Autodesk Fusion 360 part; units mm, degrees
(part 9 of 12)
sketch "草图30" plane through (71.5001, 0.0001, 0) normal (1, 0.000001, 0) x (-0.000001, 1, 0)
  line L0 (-74.9988, 0) -> (161.4999, 0)
  line L1 (161.4999, 0) -> (161.4999, 250)
  line L2 (161.4999, 250) -> (-74.9988, 250)
  line L3 (-74.9988, 250) -> (-74.9988, 0)
  line L4 (-64.9988, 15) -> (-69.3289, 12.5)
  line L5 (-69.3289, 12.5) -> (-69.3289, 7.5)
  line L6 (-69.3289, 7.5) -> (-64.9988, 5)
  line L7 (-64.9988, 5) -> (-60.6687, 7.5)
  line L8 (-60.6687, 7.5) -> (-60.6687, 12.5)
  line L9 (-60.6687, 12.5) -> (-64.9988, 15)
  line L10 (-54.3385, 15) -> (-58.6687, 12.5)
  line L11 (-58.6687, 12.5) -> (-58.6687, 7.5)
  line L12 (-58.6687, 7.5) -> (-54.3385, 5)
  line L13 (-54.3385, 5) -> (-50.0084, 7.5)
  line L14 (-50.0084, 7.5) -> (-50.0084, 12.5)
  line L15 (-50.0084, 12.5) -> (-54.3385, 15)
  line L16 (-43.6783, 15) -> (-48.0084, 12.5)
  line L17 (-48.0084, 12.5) -> (-48.0084, 7.5)
  line L18 (-48.0084, 7.5) -> (-43.6783, 5)
  line L19 (-43.6783, 5) -> (-39.3482, 7.5)
  line L20 (-39.3482, 7.5) -> (-39.3482, 12.5)
  line L21 (-39.3482, 12.5) -> (-43.6783, 15)
  line L22 (-33.018, 15) -> (-37.3482, 12.5)
  line L23 (-37.3482, 12.5) -> (-37.3482, 7.5)
  line L24 (-37.3482, 7.5) -> (-33.018, 5)
  line L25 (-33.018, 5) -> (-28.6879, 7.5)
  line L26 (-28.6879, 7.5) -> (-28.6879, 12.5)
  line L27 (-28.6879, 12.5) -> (-33.018, 15)
  line L28 (-22.3578, 15) -> (-26.6879, 12.5)
  line L29 (-26.6879, 12.5) -> (-26.6879, 7.5)
  line L30 (-26.6879, 7.5) -> (-22.3578, 5)
  line L31 (-22.3578, 5) -> (-18.0277, 7.5)
  line L32 (-18.0277, 7.5) -> (-18.0277, 12.5)
  line L33 (-18.0277, 12.5) -> (-22.3578, 15)
  line L34 (-11.6975, 15) -> (-16.0277, 12.5)
  line L35 (-16.0277, 12.5) -> (-16.0277, 7.5)
  line L36 (-16.0277, 7.5) -> (-11.6975, 5)
  line L37 (-11.6975, 5) -> (-7.3674, 7.5)
  line L38 (-7.3674, 7.5) -> (-7.3674, 12.5)
  line L39 (-7.3674, 12.5) -> (-11.6975, 15)
  line L40 (-1.0373, 15) -> (-5.3674, 12.5)
  line L41 (-5.3674, 12.5) -> (-5.3674, 7.5)
  line L42 (-5.3674, 7.5) -> (-1.0373, 5)
  line L43 (-1.0373, 5) -> (3.2929, 7.5)
  line L44 (3.2929, 7.5) -> (3.2929, 12.5)
  line L45 (3.2929, 12.5) -> (-1.0373, 15)
  line L46 (9.623, 15) -> (5.2929, 12.5)
  line L47 (5.2929, 12.5) -> (5.2929, 7.5)
  line L48 (5.2929, 7.5) -> (9.623, 5)
  line L49 (9.623, 5) -> (13.9531, 7.5)
  line L50 (13.9531, 7.5) -> (13.9531, 12.5)
  line L51 (13.9531, 12.5) -> (9.623, 15)
  line L52 (20.2832, 15) -> (15.9531, 12.5)
  line L53 (15.9531, 12.5) -> (15.9531, 7.5)
  line L54 (15.9531, 7.5) -> (20.2832, 5)
  line L55 (20.2832, 5) -> (24.6134, 7.5)
  line L56 (24.6134, 7.5) -> (24.6134, 12.5)
  line L57 (24.6134, 12.5) -> (20.2832, 15)
  line L58 (30.9435, 15) -> (26.6134, 12.5)
  line L59 (26.6134, 12.5) -> (26.6134, 7.5)
  line L60 (26.6134, 7.5) -> (30.9435, 5)
  line L61 (30.9435, 5) -> (35.2736, 7.5)
  line L62 (35.2736, 7.5) -> (35.2736, 12.5)
  line L63 (35.2736, 12.5) -> (30.9435, 15)
  line L64 (41.6037, 15) -> (37.2736, 12.5)
  line L65 (37.2736, 12.5) -> (37.2736, 7.5)
  line L66 (37.2736, 7.5) -> (41.6037, 5)
  line L67 (41.6037, 5) -> (45.9339, 7.5)
  line L68 (45.9339, 7.5) -> (45.9339, 12.5)
  line L69 (45.9339, 12.5) -> (41.6037, 15)
  line L70 (52.264, 15) -> (47.9339, 12.5)
  line L71 (47.9339, 12.5) -> (47.9339, 7.5)
  line L72 (47.9339, 7.5) -> (52.264, 5)
  line L73 (52.264, 5) -> (56.5941, 7.5)
  line L74 (56.5941, 7.5) -> (56.5941, 12.5)
  line L75 (56.5941, 12.5) -> (52.264, 15)
  line L76 (62.9242, 15) -> (58.5941, 12.5)
  line L77 (58.5941, 12.5) -> (58.5941, 7.5)
  line L78 (58.5941, 7.5) -> (62.9242, 5)
  line L79 (62.9242, 5) -> (67.2544, 7.5)
  line L80 (67.2544, 7.5) -> (67.2544, 12.5)
  line L81 (67.2544, 12.5) -> (62.9242, 15)
  line L82 (73.5845, 15) -> (69.2544, 12.5)
  line L83 (69.2544, 12.5) -> (69.2544, 7.5)
  line L84 (69.2544, 7.5) -> (73.5845, 5)
  line L85 (73.5845, 5) -> (77.9146, 7.5)
  line L86 (77.9146, 7.5) -> (77.9146, 12.5)
  line L87 (77.9146, 12.5) -> (73.5845, 15)
  line L88 (84.2448, 15) -> (79.9146, 12.5)
  line L89 (79.9146, 12.5) -> (79.9146, 7.5)
  line L90 (79.9146, 7.5) -> (84.2448, 5)
  line L91 (84.2448, 5) -> (88.5749, 7.5)
  line L92 (88.5749, 7.5) -> (88.5749, 12.5)
  line L93 (88.5749, 12.5) -> (84.2448, 15)
  line L94 (94.905, 15) -> (90.5749, 12.5)
  line L95 (90.5749, 12.5) -> (90.5749, 7.5)
  line L96 (90.5749, 7.5) -> (94.905, 5)
  line L97 (94.905, 5) -> (99.2351, 7.5)
  line L98 (99.2351, 7.5) -> (99.2351, 12.5)
  line L99 (99.2351, 12.5) -> (94.905, 15)
  line L100 (105.5653, 15) -> (101.2351, 12.5)
  line L101 (101.2351, 12.5) -> (101.2351, 7.5)
  line L102 (101.2351, 7.5) -> (105.5653, 5)
  line L103 (105.5653, 5) -> (109.8954, 7.5)
  line L104 (109.8954, 7.5) -> (109.8954, 12.5)
  line L105 (109.8954, 12.5) -> (105.5653, 15)
  line L106 (116.2255, 15) -> (111.8954, 12.5)
  line L107 (111.8954, 12.5) -> (111.8954, 7.5)
  line L108 (111.8954, 7.5) -> (116.2255, 5)
  line L109 (116.2255, 5) -> (120.5556, 7.5)
  line L110 (120.5556, 7.5) -> (120.5556, 12.5)
  line L111 (120.5556, 12.5) -> (116.2255, 15)
  line L112 (126.8858, 15) -> (122.5556, 12.5)
  line L113 (122.5556, 12.5) -> (122.5556, 7.5)
  line L114 (122.5556, 7.5) -> (126.8858, 5)
  line L115 (126.8858, 5) -> (131.2159, 7.5)
  line L116 (131.2159, 7.5) -> (131.2159, 12.5)
  line L117 (131.2159, 12.5) -> (126.8858, 15)
  line L118 (137.546, 15) -> (133.2159, 12.5)
  line L119 (133.2159, 12.5) -> (133.2159, 7.5)
  line L120 (133.2159, 7.5) -> (137.546, 5)
  line L121 (137.546, 5) -> (141.8762, 7.5)
  line L122 (141.8762, 7.5) -> (141.8762, 12.5)
  line L123 (141.8762, 12.5) -> (137.546, 15)
  line L124 (148.2063, 15) -> (143.8762, 12.5)
  line L125 (143.8762, 12.5) -> (143.8762, 7.5)
  line L126 (143.8762, 7.5) -> (148.2063, 5)
  line L127 (148.2063, 5) -> (152.5364, 7.5)
  line L128 (152.5364, 7.5) -> (152.5364, 12.5)
  line L129 (152.5364, 12.5) -> (148.2063, 15)
  line L130 (-59.6687, 24.2321) -> (-63.9988, 21.7321)
  line L131 (-63.9988, 21.7321) -> (-63.9988, 16.7321)
  line L132 (-63.9988, 16.7321) -> (-59.6687, 14.2321)
  line L133 (-59.6687, 14.2321) -> (-55.3385, 16.7321)
  line L134 (-55.3385, 16.7321) -> (-55.3385, 21.7321)
  line L135 (-55.3385, 21.7321) -> (-59.6687, 24.2321)
  line L136 (-49.0084, 24.2321) -> (-53.3385, 21.7321)
  line L137 (-53.3385, 21.7321) -> (-53.3385, 16.7321)
  line L138 (-53.3385, 16.7321) -> (-49.0084, 14.2321)
  line L139 (-49.0084, 14.2321) -> (-44.6783, 16.7321)
  line L140 (-44.6783, 16.7321) -> (-44.6783, 21.7321)
  line L141 (-44.6783, 21.7321) -> (-49.0084, 24.2321)
  line L142 (-38.3482, 24.2321) -> (-42.6783, 21.7321)
  line L143 (-42.6783, 21.7321) -> (-42.6783, 16.7321)
  line L144 (-42.6783, 16.7321) -> (-38.3482, 14.2321)
  line L145 (-38.3482, 14.2321) -> (-34.018, 16.7321)
  line L146 (-34.018, 16.7321) -> (-34.018, 21.7321)
  line L147 (-34.018, 21.7321) -> (-38.3482, 24.2321)
  line L148 (-27.6879, 24.2321) -> (-32.018, 21.7321)
  line L149 (-32.018, 21.7321) -> (-32.018, 16.7321)
  line L150 (-32.018, 16.7321) -> (-27.6879, 14.2321)
  line L151 (-27.6879, 14.2321) -> (-23.3578, 16.7321)
  line L152 (-23.3578, 16.7321) -> (-23.3578, 21.7321)
  line L153 (-23.3578, 21.7321) -> (-27.6879, 24.2321)
  line L154 (-17.0277, 24.2321) -> (-21.3578, 21.7321)
  line L155 (-21.3578, 21.7321) -> (-21.3578, 16.7321)
  line L156 (-21.3578, 16.7321) -> (-17.0277, 14.2321)
  line L157 (-17.0277, 14.2321) -> (-12.6975, 16.7321)
  line L158 (-12.6975, 16.7321) -> (-12.6975, 21.7321)
  line L159 (-12.6975, 21.7321) -> (-17.0277, 24.2321)
  line L160 (-6.3674, 24.2321) -> (-10.6975, 21.7321)
  line L161 (-10.6975, 21.7321) -> (-10.6975, 16.7321)
  line L162 (-10.6975, 16.7321) -> (-6.3674, 14.2321)
  line L163 (-6.3674, 14.2321) -> (-2.0373, 16.7321)
  line L164 (-2.0373, 16.7321) -> (-2.0373, 21.7321)
  line L165 (-2.0373, 21.7321) -> (-6.3674, 24.2321)
  line L166 (4.2929, 24.2321) -> (-0.0373, 21.7321)
  line L167 (-0.0373, 21.7321) -> (-0.0373, 16.7321)
  line L168 (-0.0373, 16.7321) -> (4.2929, 14.2321)
  line L169 (4.2929, 14.2321) -> (8.623, 16.7321)
  line L170 (8.623, 16.7321) -> (8.623, 21.7321)
  line L171 (8.623, 21.7321) -> (4.2929, 24.2321)
  line L172 (14.9531, 24.2321) -> (10.623, 21.7321)
  line L173 (10.623, 21.7321) -> (10.623, 16.7321)
  line L174 (10.623, 16.7321) -> (14.9531, 14.2321)
  line L175 (14.9531, 14.2321) -> (19.2832, 16.7321)
  line L176 (19.2832, 16.7321) -> (19.2832, 21.7321)
  line L177 (19.2832, 21.7321) -> (14.9531, 24.2321)
  line L178 (25.6134, 24.2321) -> (21.2832, 21.7321)
  line L179 (21.2832, 21.7321) -> (21.2832, 16.7321)
  line L180 (21.2832, 16.7321) -> (25.6134, 14.2321)
  line L181 (25.6134, 14.2321) -> (29.9435, 16.7321)
  line L182 (29.9435, 16.7321) -> (29.9435, 21.7321)
  line L183 (29.9435, 21.7321) -> (25.6134, 24.2321)
  line L184 (36.2736, 24.2321) -> (31.9435, 21.7321)
  line L185 (31.9435, 21.7321) -> (31.9435, 16.7321)
  line L186 (31.9435, 16.7321) -> (36.2736, 14.2321)
  line L187 (36.2736, 14.2321) -> (40.6037, 16.7321)
  line L188 (40.6037, 16.7321) -> (40.6037, 21.7321)
  line L189 (40.6037, 21.7321) -> (36.2736, 24.2321)
  line L190 (46.9339, 24.2321) -> (42.6037, 21.7321)
  line L191 (42.6037, 21.7321) -> (42.6037, 16.7321)
  line L192 (42.6037, 16.7321) -> (46.9339, 14.2321)
  line L193 (46.9339, 14.2321) -> (51.264, 16.7321)
  line L194 (51.264, 16.7321) -> (51.264, 21.7321)
  line L195 (51.264, 21.7321) -> (46.9339, 24.2321)
  line L196 (57.5941, 24.2321) -> (53.264, 21.7321)
  line L197 (53.264, 21.7321) -> (53.264, 16.7321)
  line L198 (53.264, 16.7321) -> (57.5941, 14.2321)
  line L199 (57.5941, 14.2321) -> (61.9242, 16.7321)
  line L200 (61.9242, 16.7321) -> (61.9242, 21.7321)
  line L201 (61.9242, 21.7321) -> (57.5941, 24.2321)
  line L202 (68.2544, 24.2321) -> (63.9242, 21.7321)
  line L203 (63.9242, 21.7321) -> (63.9242, 16.7321)
  line L204 (63.9242, 16.7321) -> (68.2544, 14.2321)
  line L205 (68.2544, 14.2321) -> (72.5845, 16.7321)
  line L206 (72.5845, 16.7321) -> (72.5845, 21.7321)
  line L207 (72.5845, 21.7321) -> (68.2544, 24.2321)
  line L208 (78.9146, 24.2321) -> (74.5845, 21.7321)
  line L209 (74.5845, 21.7321) -> (74.5845, 16.7321)
  line L210 (74.5845, 16.7321) -> (78.9146, 14.2321)
  line L211 (78.9146, 14.2321) -> (83.2448, 16.7321)
  line L212 (83.2448, 16.7321) -> (83.2448, 21.7321)
  line L213 (83.2448, 21.7321) -> (78.9146, 24.2321)
  line L214 (89.5749, 24.2321) -> (85.2448, 21.7321)
  line L215 (85.2448, 21.7321) -> (85.2448, 16.7321)
  line L216 (85.2448, 16.7321) -> (89.5749, 14.2321)
  line L217 (89.5749, 14.2321) -> (93.905, 16.7321)
  line L218 (93.905, 16.7321) -> (93.905, 21.7321)
  line L219 (93.905, 21.7321) -> (89.5749, 24.2321)
  line L220 (100.2351, 24.2321) -> (95.905, 21.7321)
  line L221 (95.905, 21.7321) -> (95.905, 16.7321)
  line L222 (95.905, 16.7321) -> (100.2351, 14.2321)
  line L223 (100.2351, 14.2321) -> (104.5653, 16.7321)
  line L224 (104.5653, 16.7321) -> (104.5653, 21.7321)
  line L225 (104.5653, 21.7321) -> (100.2351, 24.2321)
  line L226 (110.8954, 24.2321) -> (106.5653, 21.7321)
  line L227 (106.5653, 21.7321) -> (106.5653, 16.7321)
  line L228 (106.5653, 16.7321) -> (110.8954, 14.2321)
  line L229 (110.8954, 14.2321) -> (115.2255, 16.7321)
  line L230 (115.2255, 16.7321) -> (115.2255, 21.7321)
  line L231 (115.2255, 21.7321) -> (110.8954, 24.2321)
  line L232 (121.5556, 24.2321) -> (117.2255, 21.7321)
  line L233 (117.2255, 21.7321) -> (117.2255, 16.7321)
  line L234 (117.2255, 16.7321) -> (121.5556, 14.2321)
  line L235 (121.5556, 14.2321) -> (125.8858, 16.7321)
  line L236 (125.8858, 16.7321) -> (125.8858, 21.7321)
  line L237 (125.8858, 21.7321) -> (121.5556, 24.2321)
  line L238 (132.2159, 24.2321) -> (127.8858, 21.7321)
  line L239 (127.8858, 21.7321) -> (127.8858, 16.7321)
  line L240 (127.8858, 16.7321) -> (132.2159, 14.2321)
  line L241 (132.2159, 14.2321) -> (136.546, 16.7321)
  line L242 (136.546, 16.7321) -> (136.546, 21.7321)
  line L243 (136.546, 21.7321) -> (132.2159, 24.2321)
  line L244 (142.8762, 24.2321) -> (138.546, 21.7321)
  line L245 (138.546, 21.7321) -> (138.546, 16.7321)
  line L246 (138.546, 16.7321) -> (142.8762, 14.2321)
  line L247 (142.8762, 14.2321) -> (147.2063, 16.7321)
  line L248 (147.2063, 16.7321) -> (147.2063, 21.7321)
  line L249 (147.2063, 21.7321) -> (142.8762, 24.2321)
  line L250 (-64.9988, 33.4641) -> (-69.3289, 30.9641)
  line L251 (-69.3289, 30.9641) -> (-69.3289, 25.9641)
  line L252 (-69.3289, 25.9641) -> (-64.9988, 23.4641)
  line L253 (-64.9988, 23.4641) -> (-60.6687, 25.9641)
  line L254 (-60.6687, 25.9641) -> (-60.6687, 30.9641)
  line L255 (-60.6687, 30.9641) -> (-64.9988, 33.4641)
  line L256 (-54.3385, 33.4641) -> (-58.6687, 30.9641)
  line L257 (-58.6687, 30.9641) -> (-58.6687, 25.9641)
  line L258 (-58.6687, 25.9641) -> (-54.3385, 23.4641)
  line L259 (-54.3385, 23.4641) -> (-50.0084, 25.9641)
  line L260 (-50.0084, 25.9641) -> (-50.0084, 30.9641)
  line L261 (-50.0084, 30.9641) -> (-54.3385, 33.4641)
  line L262 (-43.6783, 33.4641) -> (-48.0084, 30.9641)
  line L263 (-48.0084, 30.9641) -> (-48.0084, 25.9641)
  line L264 (-48.0084, 25.9641) -> (-43.6783, 23.4641)
  line L265 (-43.6783, 23.4641) -> (-39.3482, 25.9641)
  line L266 (-39.3482, 25.9641) -> (-39.3482, 30.9641)
  line L267 (-39.3482, 30.9641) -> (-43.6783, 33.4641)
  line L268 (-33.018, 33.4641) -> (-37.3482, 30.9641)
  line L269 (-37.3482, 30.9641) -> (-37.3482, 25.9641)
  line L270 (-37.3482, 25.9641) -> (-33.018, 23.4641)
  line L271 (-33.018, 23.4641) -> (-28.6879, 25.9641)
  line L272 (-28.6879, 25.9641) -> (-28.6879, 30.9641)
  line L273 (-28.6879, 30.9641) -> (-33.018, 33.4641)
  line L274 (-22.3578, 33.4641) -> (-26.6879, 30.9641)
  line L275 (-26.6879, 30.9641) -> (-26.6879, 25.9641)
  line L276 (-26.6879, 25.9641) -> (-22.3578, 23.4641)
  line L277 (-22.3578, 23.4641) -> (-18.0277, 25.9641)
  line L278 (-18.0277, 25.9641) -> (-18.0277, 30.9641)
  line L279 (-18.0277, 30.9641) -> (-22.3578, 33.4641)
  line L280 (-11.6975, 33.4641) -> (-16.0277, 30.9641)
  line L281 (-16.0277, 30.9641) -> (-16.0277, 25.9641)
  line L282 (-16.0277, 25.9641) -> (-11.6975, 23.4641)
  line L283 (-11.6975, 23.4641) -> (-7.3674, 25.9641)
  line L284 (-7.3674, 25.9641) -> (-7.3674, 30.9641)
  line L285 (-7.3674, 30.9641) -> (-11.6975, 33.4641)
  line L286 (-1.0373, 33.4641) -> (-5.3674, 30.9641)
  line L287 (-5.3674, 30.9641) -> (-5.3674, 25.9641)
  line L288 (-5.3674, 25.9641) -> (-1.0373, 23.4641)
  line L289 (-1.0373, 23.4641) -> (3.2929, 25.9641)
  line L290 (3.2929, 25.9641) -> (3.2929, 30.9641)
  line L291 (3.2929, 30.9641) -> (-1.0373, 33.4641)
  line L292 (9.623, 33.4641) -> (5.2929, 30.9641)
  line L293 (5.2929, 30.9641) -> (5.2929, 25.9641)
  line L294 (5.2929, 25.9641) -> (9.623, 23.4641)
  line L295 (9.623, 23.4641) -> (13.9531, 25.9641)
  line L296 (13.9531, 25.9641) -> (13.9531, 30.9641)
  line L297 (13.9531, 30.9641) -> (9.623, 33.4641)
  line L298 (20.2832, 33.4641) -> (15.9531, 30.9641)
  line L299 (15.9531, 30.9641) -> (15.9531, 25.9641)
  line L300 (15.9531, 25.9641) -> (20.2832, 23.4641)
  line L301 (20.2832, 23.4641) -> (24.6134, 25.9641)
  line L302 (24.6134, 25.9641) -> (24.6134, 30.9641)
  line L303 (24.6134, 30.9641) -> (20.2832, 33.4641)
  line L304 (30.9435, 33.4641) -> (26.6134, 30.9641)
  line L305 (26.6134, 30.9641) -> (26.6134, 25.9641)
  line L306 (26.6134, 25.9641) -> (30.9435, 23.4641)
  line L307 (30.9435, 23.4641) -> (35.2736, 25.9641)
  line L308 (35.2736, 25.9641) -> (35.2736, 30.9641)
  line L309 (35.2736, 30.9641) -> (30.9435, 33.4641)
  line L310 (41.6037, 33.4641) -> (37.2736, 30.9641)
  line L311 (37.2736, 30.9641) -> (37.2736, 25.9641)
  line L312 (37.2736, 25.9641) -> (41.6037, 23.4641)
  line L313 (41.6037, 23.4641) -> (45.9339, 25.9641)
  line L314 (45.9339, 25.9641) -> (45.9339, 30.9641)
  line L315 (45.9339, 30.9641) -> (41.6037, 33.4641)
  line L316 (52.264, 33.4641) -> (47.9339, 30.9641)
  line L317 (47.9339, 30.9641) -> (47.9339, 25.9641)
  line L318 (47.9339, 25.9641) -> (52.264, 23.4641)
  line L319 (52.264, 23.4641) -> (56.5941, 25.9641)
  line L320 (56.5941, 25.9641) -> (56.5941, 30.9641)
  line L321 (56.5941, 30.9641) -> (52.264, 33.4641)
  line L322 (62.9242, 33.4641) -> (58.5941, 30.9641)
  line L323 (58.5941, 30.9641) -> (58.5941, 25.9641)
  line L324 (58.5941, 25.9641) -> (62.9242, 23.4641)
  line L325 (62.9242, 23.4641) -> (67.2544, 25.9641)
  line L326 (67.2544, 25.9641) -> (67.2544, 30.9641)
  line L327 (67.2544, 30.9641) -> (62.9242, 33.4641)
  line L328 (73.5845, 33.4641) -> (69.2544, 30.9641)
  line L329 (69.2544, 30.9641) -> (69.2544, 25.9641)
  line L330 (69.2544, 25.9641) -> (73.5845, 23.4641)
  line L331 (73.5845, 23.4641) -> (77.9146, 25.9641)
  line L332 (77.9146, 25.9641) -> (77.9146, 30.9641)
  line L333 (77.9146, 30.9641) -> (73.5845, 33.4641)
  line L334 (84.2448, 33.4641) -> (79.9146, 30.9641)
  line L335 (79.9146, 30.9641) -> (79.9146, 25.9641)
  line L336 (79.9146, 25.9641) -> (84.2448, 23.4641)
  line L337 (84.2448, 23.4641) -> (88.5749, 25.9641)
  line L338 (88.5749, 25.9641) -> (88.5749, 30.9641)
  line L339 (88.5749, 30.9641) -> (84.2448, 33.4641)
  line L340 (94.905, 33.4641) -> (90.5749, 30.9641)
  line L341 (90.5749, 30.9641) -> (90.5749, 25.9641)
  line L342 (90.5749, 25.9641) -> (94.905, 23.4641)
  line L343 (94.905, 23.4641) -> (99.2351, 25.9641)
  line L344 (99.2351, 25.9641) -> (99.2351, 30.9641)
  line L345 (99.2351, 30.9641) -> (94.905, 33.4641)
  line L346 (105.5653, 33.4641) -> (101.2351, 30.9641)
  line L347 (101.2351, 30.9641) -> (101.2351, 25.9641)
  line L348 (101.2351, 25.9641) -> (105.5653, 23.4641)
  line L349 (105.5653, 23.4641) -> (109.8954, 25.9641)
  line L350 (109.8954, 25.9641) -> (109.8954, 30.9641)
  line L351 (109.8954, 30.9641) -> (105.5653, 33.4641)
  line L352 (116.2255, 33.4641) -> (111.8954, 30.9641)
  line L353 (111.8954, 30.9641) -> (111.8954, 25.9641)
  line L354 (111.8954, 25.9641) -> (116.2255, 23.4641)
  line L355 (116.2255, 23.4641) -> (120.5556, 25.9641)
  line L356 (120.5556, 25.9641) -> (120.5556, 30.9641)
  line L357 (120.5556, 30.9641) -> (116.2255, 33.4641)
  line L358 (126.8858, 33.4641) -> (122.5556, 30.9641)
  line L359 (122.5556, 30.9641) -> (122.5556, 25.9641)
  line L360 (122.5556, 25.9641) -> (126.8858, 23.4641)
  line L361 (126.8858, 23.4641) -> (131.2159, 25.9641)
  line L362 (131.2159, 25.9641) -> (131.2159, 30.9641)
  line L363 (131.2159, 30.9641) -> (126.8858, 33.4641)
  line L364 (137.546, 33.4641) -> (133.2159, 30.9641)
  line L365 (133.2159, 30.9641) -> (133.2159, 25.9641)
  line L366 (133.2159, 25.9641) -> (137.546, 23.4641)
  line L367 (137.546, 23.4641) -> (141.8762, 25.9641)
  line L368 (141.8762, 25.9641) -> (141.8762, 30.9641)
  line L369 (141.8762, 30.9641) -> (137.546, 33.4641)
  line L370 (148.2063, 33.4641) -> (143.8762, 30.9641)
  line L371 (143.8762, 30.9641) -> (143.8762, 25.9641)
  line L372 (143.8762, 25.9641) -> (148.2063, 23.4641)
  line L373 (148.2063, 23.4641) -> (152.5364, 25.9641)
  line L374 (152.5364, 25.9641) -> (152.5364, 30.9641)
  line L375 (152.5364, 30.9641) -> (148.2063, 33.4641)
  line L376 (-59.6687, 42.6962) -> (-63.9988, 40.1962)
  line L377 (-63.9988, 40.1962) -> (-63.9988, 35.1962)
  line L378 (-63.9988, 35.1962) -> (-59.6687, 32.6962)
  line L379 (-59.6687, 32.6962) -> (-55.3385, 35.1962)
  line L380 (-55.3385, 35.1962) -> (-55.3385, 40.1962)
  line L381 (-55.3385, 40.1962) -> (-59.6687, 42.6962)
  line L382 (-49.0084, 42.6962) -> (-53.3385, 40.1962)
  line L383 (-53.3385, 40.1962) -> (-53.3385, 35.1962)
  line L384 (-53.3385, 35.1962) -> (-49.0084, 32.6962)
  line L385 (-49.0084, 32.6962) -> (-44.6783, 35.1962)
  line L386 (-44.6783, 35.1962) -> (-44.6783, 40.1962)
  line L387 (-44.6783, 40.1962) -> (-49.0084, 42.6962)
  line L388 (-38.3482, 42.6962) -> (-42.6783, 40.1962)
  line L389 (-42.6783, 40.1962) -> (-42.6783, 35.1962)
  line L390 (-42.6783, 35.1962) -> (-38.3482, 32.6962)
  line L391 (-38.3482, 32.6962) -> (-34.018, 35.1962)
  line L392 (-34.018, 35.1962) -> (-34.018, 40.1962)
  line L393 (-34.018, 40.1962) -> (-38.3482, 42.6962)
  line L394 (-27.6879, 42.6962) -> (-32.018, 40.1962)
  line L395 (-32.018, 40.1962) -> (-32.018, 35.1962)
  line L396 (-32.018, 35.1962) -> (-27.6879, 32.6962)
  line L397 (-27.6879, 32.6962) -> (-23.3578, 35.1962)
  line L398 (-23.3578, 35.1962) -> (-23.3578, 40.1962)
  line L399 (-23.3578, 40.1962) -> (-27.6879, 42.6962)
  line L400 (-17.0277, 42.6962) -> (-21.3578, 40.1962)
  line L401 (-21.3578, 40.1962) -> (-21.3578, 35.1962)
  line L402 (-21.3578, 35.1962) -> (-17.0277, 32.6962)
  line L403 (-17.0277, 32.6962) -> (-12.6975, 35.1962)
  line L404 (-12.6975, 35.1962) -> (-12.6975, 40.1962)
  line L405 (-12.6975, 40.1962) -> (-17.0277, 42.6962)
  line L406 (-6.3674, 42.6962) -> (-10.6975, 40.1962)
  line L407 (-10.6975, 40.1962) -> (-10.6975, 35.1962)
  line L408 (-10.6975, 35.1962) -> (-6.3674, 32.6962)
  line L409 (-6.3674, 32.6962) -> (-2.0373, 35.1962)
  line L410 (-2.0373, 35.1962) -> (-2.0373, 40.1962)
  line L411 (-2.0373, 40.1962) -> (-6.3674, 42.6962)
  line L412 (4.2929, 42.6962) -> (-0.0373, 40.1962)
  line L413 (-0.0373, 40.1962) -> (-0.0373, 35.1962)
  line L414 (-0.0373, 35.1962) -> (4.2929, 32.6962)
  line L415 (4.2929, 32.6962) -> (8.623, 35.1962)
  line L416 (8.623, 35.1962) -> (8.623, 40.1962)
  line L417 (8.623, 40.1962) -> (4.2929, 42.6962)
  line L418 (14.9531, 42.6962) -> (10.623, 40.1962)
  line L419 (10.623, 40.1962) -> (10.623, 35.1962)
  line L420 (10.623, 35.1962) -> (14.9531, 32.6962)
  line L421 (14.9531, 32.6962) -> (19.2832, 35.1962)
  line L422 (19.2832, 35.1962) -> (19.2832, 40.1962)
  line L423 (19.2832, 40.1962) -> (14.9531, 42.6962)
  line L424 (25.6134, 42.6962) -> (21.2832, 40.1962)
  line L425 (21.2832, 40.1962) -> (21.2832, 35.1962)
  line L426 (21.2832, 35.1962) -> (25.6134, 32.6962)
  line L427 (25.6134, 32.6962) -> (29.9435, 35.1962)
  line L428 (29.9435, 35.1962) -> (29.9435, 40.1962)
  line L429 (29.9435, 40.1962) -> (25.6134, 42.6962)
  line L430 (36.2736, 42.6962) -> (31.9435, 40.1962)
  line L431 (31.9435, 40.1962) -> (31.9435, 35.1962)
  line L432 (31.9435, 35.1962) -> (36.2736, 32.6962)
  line L433 (36.2736, 32.6962) -> (40.6037, 35.1962)
  line L434 (40.6037, 35.1962) -> (40.6037, 40.1962)
  line L435 (40.6037, 40.1962) -> (36.2736, 42.6962)
  line L436 (46.9339, 42.6962) -> (42.6037, 40.1962)
  line L437 (42.6037, 40.1962) -> (42.6037, 35.1962)
  line L438 (42.6037, 35.1962) -> (46.9339, 32.6962)
  line L439 (46.9339, 32.6962) -> (51.264, 35.1962)
  line L440 (51.264, 35.1962) -> (51.264, 40.1962)
  line L441 (51.264, 40.1962) -> (46.9339, 42.6962)
  line L442 (57.5941, 42.6962) -> (53.264, 40.1962)
  line L443 (53.264, 40.1962) -> (53.264, 35.1962)
  line L444 (53.264, 35.1962) -> (57.5941, 32.6962)
  line L445 (57.5941, 32.6962) -> (61.9242, 35.1962)
  line L446 (61.9242, 35.1962) -> (61.9242, 40.1962)
  line L447 (61.9242, 40.1962) -> (57.5941, 42.6962)
  line L448 (68.2544, 42.6962) -> (63.9242, 40.1962)
  line L449 (63.9242, 40.1962) -> (63.9242, 35.1962)
  line L450 (63.9242, 35.1962) -> (68.2544, 32.6962)
  line L451 (68.2544, 32.6962) -> (72.5845, 35.1962)
  line L452 (72.5845, 35.1962) -> (72.5845, 40.1962)
  line L453 (72.5845, 40.1962) -> (68.2544, 42.6962)
  line L454 (78.9146, 42.6962) -> (74.5845, 40.1962)
  line L455 (74.5845, 40.1962) -> (74.5845, 35.1962)
  line L456 (74.5845, 35.1962) -> (78.9146, 32.6962)
  line L457 (78.9146, 32.6962) -> (83.2448, 35.1962)
  line L458 (83.2448, 35.1962) -> (83.2448, 40.1962)
  line L459 (83.2448, 40.1962) -> (78.9146, 42.6962)
  line L460 (89.5749, 42.6962) -> (85.2448, 40.1962)
  line L461 (85.2448, 40.1962) -> (85.2448, 35.1962)
  line L462 (85.2448, 35.1962) -> (89.5749, 32.6962)
  line L463 (89.5749, 32.6962) -> (93.905, 35.1962)
  line L464 (93.905, 35.1962) -> (93.905, 40.1962)
  line L465 (93.905, 40.1962) -> (89.5749, 42.6962)
  line L466 (100.2351, 42.6962) -> (95.905, 40.1962)
  line L467 (95.905, 40.1962) -> (95.905, 35.1962)
  line L468 (95.905, 35.1962) -> (100.2351, 32.6962)
  line L469 (100.2351, 32.6962) -> (104.5653, 35.1962)
  line L470 (104.5653, 35.1962) -> (104.5653, 40.1962)
  line L471 (104.5653, 40.1962) -> (100.2351, 42.6962)
  line L472 (110.8954, 42.6962) -> (106.5653, 40.1962)
  line L473 (106.5653, 40.1962) -> (106.5653, 35.1962)
  line L474 (106.5653, 35.1962) -> (110.8954, 32.6962)
  line L475 (110.8954, 32.6962) -> (115.2255, 35.1962)
  line L476 (115.2255, 35.1962) -> (115.2255, 40.1962)
  line L477 (115.2255, 40.1962) -> (110.8954, 42.6962)
  line L478 (121.5556, 42.6962) -> (117.2255, 40.1962)
  line L479 (117.2255, 40.1962) -> (117.2255, 35.1962)
  line L480 (117.2255, 35.1962) -> (121.5556, 32.6962)
  line L481 (121.5556, 32.6962) -> (125.8858, 35.1962)
  line L482 (125.8858, 35.1962) -> (125.8858, 40.1962)
  line L483 (125.8858, 40.1962) -> (121.5556, 42.6962)
  line L484 (132.2159, 42.6962) -> (127.8858, 40.1962)
  line L485 (127.8858, 40.1962) -> (127.8858, 35.1962)
  line L486 (127.8858, 35.1962) -> (132.2159, 32.6962)
  line L487 (132.2159, 32.6962) -> (136.546, 35.1962)
  line L488 (136.546, 35.1962) -> (136.546, 40.1962)
  line L489 (136.546, 40.1962) -> (132.2159, 42.6962)
  line L490 (142.8762, 42.6962) -> (138.546, 40.1962)
  line L491 (138.546, 40.1962) -> (138.546, 35.1962)
  line L492 (138.546, 35.1962) -> (142.8762, 32.6962)
  line L493 (142.8762, 32.6962) -> (147.2063, 35.1962)
  line L494 (147.2063, 35.1962) -> (147.2063, 40.1962)
  line L495 (147.2063, 40.1962) -> (142.8762, 42.6962)
  line L496 (-64.9988, 51.9282) -> (-69.3289, 49.4282)
  line L497 (-69.3289, 49.4282) -> (-69.3289, 44.4282)
  line L498 (-69.3289, 44.4282) -> (-64.9988, 41.9282)
  line L499 (-64.9988, 41.9282) -> (-60.6687, 44.4282)
  line L500 (-60.6687, 44.4282) -> (-60.6687, 49.4282)
  line L501 (-60.6687, 49.4282) -> (-64.9988, 51.9282)
  line L502 (-54.3385, 51.9282) -> (-58.6687, 49.4282)
  line L503 (-58.6687, 49.4282) -> (-58.6687, 44.4282)
  line L504 (-58.6687, 44.4282) -> (-54.3385, 41.9282)
  line L505 (-54.3385, 41.9282) -> (-50.0084, 44.4282)
  line L506 (-50.0084, 44.4282) -> (-50.0084, 49.4282)
  line L507 (-50.0084, 49.4282) -> (-54.3385, 51.9282)
  line L508 (-43.6783, 51.9282) -> (-48.0084, 49.4282)
  line L509 (-48.0084, 49.4282) -> (-48.0084, 44.4282)
  line L510 (-48.0084, 44.4282) -> (-43.6783, 41.9282)
  line L511 (-43.6783, 41.9282) -> (-39.3482, 44.4282)
  line L512 (-39.3482, 44.4282) -> (-39.3482, 49.4282)
  line L513 (-39.3482, 49.4282) -> (-43.6783, 51.9282)
  line L514 (-33.018, 51.9282) -> (-37.3482, 49.4282)
  line L515 (-37.3482, 49.4282) -> (-37.3482, 44.4282)
  line L516 (-37.3482, 44.4282) -> (-33.018, 41.9282)
  line L517 (-33.018, 41.9282) -> (-28.6879, 44.4282)
  line L518 (-28.6879, 44.4282) -> (-28.6879, 49.4282)
  line L519 (-28.6879, 49.4282) -> (-33.018, 51.9282)
  line L520 (-22.3578, 51.9282) -> (-26.6879, 49.4282)
  line L521 (-26.6879, 49.4282) -> (-26.6879, 44.4282)
  line L522 (-26.6879, 44.4282) -> (-22.3578, 41.9282)
  line L523 (-22.3578, 41.9282) -> (-18.0277, 44.4282)
  line L524 (-18.0277, 44.4282) -> (-18.0277, 49.4282)
  line L525 (-18.0277, 49.4282) -> (-22.3578, 51.9282)
  line L526 (-11.6975, 51.9282) -> (-16.0277, 49.4282)
  line L527 (-16.0277, 49.4282) -> (-16.0277, 44.4282)
  line L528 (-16.0277, 44.4282) -> (-11.6975, 41.9282)
  line L529 (-11.6975, 41.9282) -> (-7.3674, 44.4282)
  line L530 (-7.3674, 44.4282) -> (-7.3674, 49.4282)
  line L531 (-7.3674, 49.4282) -> (-11.6975, 51.9282)
  line L532 (-1.0373, 51.9282) -> (-5.3674, 49.4282)
  line L533 (-5.3674, 49.4282) -> (-5.3674, 44.4282)
  line L534 (-5.3674, 44.4282) -> (-1.0373, 41.9282)
  line L535 (-1.0373, 41.9282) -> (3.2929, 44.4282)
  line L536 (3.2929, 44.4282) -> (3.2929, 49.4282)
  line L537 (3.2929, 49.4282) -> (-1.0373, 51.9282)
  line L538 (9.623, 51.9282) -> (5.2929, 49.4282)
  line L539 (5.2929, 49.4282) -> (5.2929, 44.4282)
  line L540 (5.2929, 44.4282) -> (9.623, 41.9282)
  line L541 (9.623, 41.9282) -> (13.9531, 44.4282)
  line L542 (13.9531, 44.4282) -> (13.9531, 49.4282)
  line L543 (13.9531, 49.4282) -> (9.623, 51.9282)
  line L544 (20.2832, 51.9282) -> (15.9531, 49.4282)
  line L545 (15.9531, 49.4282) -> (15.9531, 44.4282)
  line L546 (15.9531, 44.4282) -> (20.2832, 41.9282)
  line L547 (20.2832, 41.9282) -> (24.6134, 44.4282)
  line L548 (24.6134, 44.4282) -> (24.6134, 49.4282)
  line L549 (24.6134, 49.4282) -> (20.2832, 51.9282)
  line L550 (30.9435, 51.9282) -> (26.6134, 49.4282)
  line L551 (26.6134, 49.4282) -> (26.6134, 44.4282)
  line L552 (26.6134, 44.4282) -> (30.9435, 41.9282)
  line L553 (30.9435, 41.9282) -> (35.2736, 44.4282)
  line L554 (35.2736, 44.4282) -> (35.2736, 49.4282)
  line L555 (35.2736, 49.4282) -> (30.9435, 51.9282)
  line L556 (41.6037, 51.9282) -> (37.2736, 49.4282)
  line L557 (37.2736, 49.4282) -> (37.2736, 44.4282)
  line L558 (37.2736, 44.4282) -> (41.6037, 41.9282)
  line L559 (41.6037, 41.9282) -> (45.9339, 44.4282)
  line L560 (45.9339, 44.4282) -> (45.9339, 49.4282)
  line L561 (45.9339, 49.4282) -> (41.6037, 51.9282)
  line L562 (52.264, 51.9282) -> (47.9339, 49.4282)
  line L563 (47.9339, 49.4282) -> (47.9339, 44.4282)
  line L564 (47.9339, 44.4282) -> (52.264, 41.9282)
  line L565 (52.264, 41.9282) -> (56.5941, 44.4282)
  line L566 (56.5941, 44.4282) -> (56.5941, 49.4282)
  line L567 (56.5941, 49.4282) -> (52.264, 51.9282)
  line L568 (62.9242, 51.9282) -> (58.5941, 49.4282)
  line L569 (58.5941, 49.4282) -> (58.5941, 44.4282)
  line L570 (58.5941, 44.4282) -> (62.9242, 41.9282)
  line L571 (62.9242, 41.9282) -> (67.2544, 44.4282)
  line L572 (67.2544, 44.4282) -> (67.2544, 49.4282)
  line L573 (67.2544, 49.4282) -> (62.9242, 51.9282)
  line L574 (73.5845, 51.9282) -> (69.2544, 49.4282)
  line L575 (69.2544, 49.4282) -> (69.2544, 44.4282)
  line L576 (69.2544, 44.4282) -> (73.5845, 41.9282)
  line L577 (73.5845, 41.9282) -> (77.9146, 44.4282)
  line L578 (77.9146, 44.4282) -> (77.9146, 49.4282)
  line L579 (77.9146, 49.4282) -> (73.5845, 51.9282)
  line L580 (84.2448, 51.9282) -> (79.9146, 49.4282)
  line L581 (79.9146, 49.4282) -> (79.9146, 44.4282)
  line L582 (79.9146, 44.4282) -> (84.2448, 41.9282)
  line L583 (84.2448, 41.9282) -> (88.5749, 44.4282)
  line L584 (88.5749, 44.4282) -> (88.5749, 49.4282)
  line L585 (88.5749, 49.4282) -> (84.2448, 51.9282)
  line L586 (94.905, 51.9282) -> (90.5749, 49.4282)
  line L587 (90.5749, 49.4282) -> (90.5749, 44.4282)
  line L588 (90.5749, 44.4282) -> (94.905, 41.9282)
  line L589 (94.905, 41.9282) -> (99.2351, 44.4282)
  line L590 (99.2351, 44.4282) -> (99.2351, 49.4282)
  line L591 (99.2351, 49.4282) -> (94.905, 51.9282)
  line L592 (105.5653, 51.9282) -> (101.2351, 49.4282)
  line L593 (101.2351, 49.4282) -> (101.2351, 44.4282)
  line L594 (101.2351, 44.4282) -> (105.5653, 41.9282)
  line L595 (105.5653, 41.9282) -> (109.8954, 44.4282)
  line L596 (109.8954, 44.4282) -> (109.8954, 49.4282)
  line L597 (109.8954, 49.4282) -> (105.5653, 51.9282)
  line L598 (116.2255, 51.9282) -> (111.8954, 49.4282)
  line L599 (111.8954, 49.4282) -> (111.8954, 44.4282)
  line L600 (111.8954, 44.4282) -> (116.2255, 41.9282)
  line L601 (116.2255, 41.9282) -> (120.5556, 44.4282)
  line L602 (120.5556, 44.4282) -> (120.5556, 49.4282)
  line L603 (120.5556, 49.4282) -> (116.2255, 51.9282)
  line L604 (126.8858, 51.9282) -> (122.5556, 49.4282)
  line L605 (122.5556, 49.4282) -> (122.5556, 44.4282)
  line L606 (122.5556, 44.4282) -> (126.8858, 41.9282)
  line L607 (126.8858, 41.9282) -> (131.2159, 44.4282)
  line L608 (131.2159, 44.4282) -> (131.2159, 49.4282)
  line L609 (131.2159, 49.4282) -> (126.8858, 51.9282)
  line L610 (137.546, 51.9282) -> (133.2159, 49.4282)
  line L611 (133.2159, 49.4282) -> (133.2159, 44.4282)
  line L612 (133.2159, 44.4282) -> (137.546, 41.9282)
  line L613 (137.546, 41.9282) -> (141.8762, 44.4282)
  line L614 (141.8762, 44.4282) -> (141.8762, 49.4282)
  line L615 (141.8762, 49.4282) -> (137.546, 51.9282)
  line L616 (148.2063, 51.9282) -> (143.8762, 49.4282)
  line L617 (143.8762, 49.4282) -> (143.8762, 44.4282)
  line L618 (143.8762, 44.4282) -> (148.2063, 41.9282)
  line L619 (148.2063, 41.9282) -> (152.5364, 44.4282)
  line L620 (152.5364, 44.4282) -> (152.5364, 49.4282)
  line L621 (152.5364, 49.4282) -> (148.2063, 51.9282)
  line L622 (-59.6687, 61.1603) -> (-63.9988, 58.6603)
  line L623 (-63.9988, 58.6603) -> (-63.9988, 53.6603)
  line L624 (-63.9988, 53.6603) -> (-59.6687, 51.1603)
  line L625 (-59.6687, 51.1603) -> (-55.3385, 53.6603)
  line L626 (-55.3385, 53.6603) -> (-55.3385, 58.6603)
  line L627 (-55.3385, 58.6603) -> (-59.6687, 61.1603)
  line L628 (-49.0084, 61.1603) -> (-53.3385, 58.6603)
  line L629 (-53.3385, 58.6603) -> (-53.3385, 53.6603)
  line L630 (-53.3385, 53.6603) -> (-49.0084, 51.1603)
  line L631 (-49.0084, 51.1603) -> (-44.6783, 53.6603)
  line L632 (-44.6783, 53.6603) -> (-44.6783, 58.6603)
  line L633 (-44.6783, 58.6603) -> (-49.0084, 61.1603)
  line L634 (-38.3482, 61.1603) -> (-42.6783, 58.6603)
  line L635 (-42.6783, 58.6603) -> (-42.6783, 53.6603)
  line L636 (-42.6783, 53.6603) -> (-38.3482, 51.1603)
  line L637 (-38.3482, 51.1603) -> (-34.018, 53.6603)
  line L638 (-34.018, 53.6603) -> (-34.018, 58.6603)
  line L639 (-34.018, 58.6603) -> (-38.3482, 61.1603)
  line L640 (-27.6879, 61.1603) -> (-32.018, 58.6603)
  line L641 (-32.018, 58.6603) -> (-32.018, 53.6603)
  line L642 (-32.018, 53.6603) -> (-27.6879, 51.1603)
  line L643 (-27.6879, 51.1603) -> (-23.3578, 53.6603)
  line L644 (-23.3578, 53.6603) -> (-23.3578, 58.6603)
  line L645 (-23.3578, 58.6603) -> (-27.6879, 61.1603)
  line L646 (-17.0277, 61.1603) -> (-21.3578, 58.6603)
  line L647 (-21.3578, 58.6603) -> (-21.3578, 53.6603)
  line L648 (-21.3578, 53.6603) -> (-17.0277, 51.1603)
  line L649 (-17.0277, 51.1603) -> (-12.6975, 53.6603)
  line L650 (-12.6975, 53.6603) -> (-12.6975, 58.6603)
  line L651 (-12.6975, 58.6603) -> (-17.0277, 61.1603)
  line L652 (-6.3674, 61.1603) -> (-10.6975, 58.6603)
  line L653 (-10.6975, 58.6603) -> (-10.6975, 53.6603)
  line L654 (-10.6975, 53.6603) -> (-6.3674, 51.1603)
  line L655 (-6.3674, 51.1603) -> (-2.0373, 53.6603)
  line L656 (-2.0373, 53.6603) -> (-2.0373, 58.6603)
  line L657 (-2.0373, 58.6603) -> (-6.3674, 61.1603)
  line L658 (4.2929, 61.1603) -> (-0.0373, 58.6603)
  line L659 (-0.0373, 58.6603) -> (-0.0373, 53.6603)
  line L660 (-0.0373, 53.6603) -> (4.2929, 51.1603)
  line L661 (4.2929, 51.1603) -> (8.623, 53.6603)
  line L662 (8.623, 53.6603) -> (8.623, 58.6603)
  line L663 (8.623, 58.6603) -> (4.2929, 61.1603)
  line L664 (14.9531, 61.1603) -> (10.623, 58.6603)
  line L665 (10.623, 58.6603) -> (10.623, 53.6603)
  line L666 (10.623, 53.6603) -> (14.9531, 51.1603)
  line L667 (14.9531, 51.1603) -> (19.2832, 53.6603)
  line L668 (19.2832, 53.6603) -> (19.2832, 58.6603)
  line L669 (19.2832, 58.6603) -> (14.9531, 61.1603)
  line L670 (25.6134, 61.1603) -> (21.2832, 58.6603)
  line L671 (21.2832, 58.6603) -> (21.2832, 53.6603)
  line L672 (21.2832, 53.6603) -> (25.6134, 51.1603)
  line L673 (25.6134, 51.1603) -> (29.9435, 53.6603)
  line L674 (29.9435, 53.6603) -> (29.9435, 58.6603)
  line L675 (29.9435, 58.6603) -> (25.6134, 61.1603)
  line L676 (36.2736, 61.1603) -> (31.9435, 58.6603)
  line L677 (31.9435, 58.6603) -> (31.9435, 53.6603)
  line L678 (31.9435, 53.6603) -> (36.2736, 51.1603)
  line L679 (36.2736, 51.1603) -> (40.6037, 53.6603)
  line L680 (40.6037, 53.6603) -> (40.6037, 58.6603)
  line L681 (40.6037, 58.6603) -> (36.2736, 61.1603)
  line L682 (46.9339, 61.1603) -> (42.6037, 58.6603)
  line L683 (42.6037, 58.6603) -> (42.6037, 53.6603)
  line L684 (42.6037, 53.6603) -> (46.9339, 51.1603)
  line L685 (46.9339, 51.1603) -> (51.264, 53.6603)
  line L686 (51.264, 53.6603) -> (51.264, 58.6603)
  line L687 (51.264, 58.6603) -> (46.9339, 61.1603)
  line L688 (57.5941, 61.1603) -> (53.264, 58.6603)
  line L689 (53.264, 58.6603) -> (53.264, 53.6603)
  line L690 (53.264, 53.6603) -> (57.5941, 51.1603)
  line L691 (57.5941, 51.1603) -> (61.9242, 53.6603)
  line L692 (61.9242, 53.6603) -> (61.9242, 58.6603)
  line L693 (61.9242, 58.6603) -> (57.5941, 61.1603)
  line L694 (68.2544, 61.1603) -> (63.9242, 58.6603)
  line L695 (63.9242, 58.6603) -> (63.9242, 53.6603)
  line L696 (63.9242, 53.6603) -> (68.2544, 51.1603)
  line L697 (68.2544, 51.1603) -> (72.5845, 53.6603)
  line L698 (72.5845, 53.6603) -> (72.5845, 58.6603)
  line L699 (72.5845, 58.6603) -> (68.2544, 61.1603)
  line L700 (78.9146, 61.1603) -> (74.5845, 58.6603)
  line L701 (74.5845, 58.6603) -> (74.5845, 53.6603)
  line L702 (74.5845, 53.6603) -> (78.9146, 51.1603)
  line L703 (78.9146, 51.1603) -> (83.2448, 53.6603)
  line L704 (83.2448, 53.6603) -> (83.2448, 58.6603)
  line L705 (83.2448, 58.6603) -> (78.9146, 61.1603)
  line L706 (89.5749, 61.1603) -> (85.2448, 58.6603)
  line L707 (85.2448, 58.6603) -> (85.2448, 53.6603)
  line L708 (85.2448, 53.6603) -> (89.5749, 51.1603)
  line L709 (89.5749, 51.1603) -> (93.905, 53.6603)
  line L710 (93.905, 53.6603) -> (93.905, 58.6603)
  line L711 (93.905, 58.6603) -> (89.5749, 61.1603)
  line L712 (100.2351, 61.1603) -> (95.905, 58.6603)
  line L713 (95.905, 58.6603) -> (95.905, 53.6603)
  line L714 (95.905, 53.6603) -> (100.2351, 51.1603)
  line L715 (100.2351, 51.1603) -> (104.5653, 53.6603)
  line L716 (104.5653, 53.6603) -> (104.5653, 58.6603)
  line L717 (104.5653, 58.6603) -> (100.2351, 61.1603)
  line L718 (110.8954, 61.1603) -> (106.5653, 58.6603)
  line L719 (106.5653, 58.6603) -> (106.5653, 53.6603)
  line L720 (106.5653, 53.6603) -> (110.8954, 51.1603)
  line L721 (110.8954, 51.1603) -> (115.2255, 53.6603)
  line L722 (115.2255, 53.6603) -> (115.2255, 58.6603)
  line L723 (115.2255, 58.6603) -> (110.8954, 61.1603)
  line L724 (121.5556, 61.1603) -> (117.2255, 58.6603)
  line L725 (117.2255, 58.6603) -> (117.2255, 53.6603)
  line L726 (117.2255, 53.6603) -> (121.5556, 51.1603)
  line L727 (121.5556, 51.1603) -> (125.8858, 53.6603)
  line L728 (125.8858, 53.6603) -> (125.8858, 58.6603)
  line L729 (125.8858, 58.6603) -> (121.5556, 61.1603)
  line L730 (132.2159, 61.1603) -> (127.8858, 58.6603)
  line L731 (127.8858, 58.6603) -> (127.8858, 53.6603)
  line L732 (127.8858, 53.6603) -> (132.2159, 51.1603)
  line L733 (132.2159, 51.1603) -> (136.546, 53.6603)
  line L734 (136.546, 53.6603) -> (136.546, 58.6603)
  line L735 (136.546, 58.6603) -> (132.2159, 61.1603)
  line L736 (142.8762, 61.1603) -> (138.546, 58.6603)
  line L737 (138.546, 58.6603) -> (138.546, 53.6603)
  line L738 (138.546, 53.6603) -> (142.8762, 51.1603)
  line L739 (142.8762, 51.1603) -> (147.2063, 53.6603)
  line L740 (147.2063, 53.6603) -> (147.2063, 58.6603)
  line L741 (147.2063, 58.6603) -> (142.8762, 61.1603)
  line L742 (-64.9988, 70.3923) -> (-69.3289, 67.8923)
  line L743 (-69.3289, 67.8923) -> (-69.3289, 62.8923)
  line L744 (-69.3289, 62.8923) -> (-64.9988, 60.3923)
  line L745 (-64.9988, 60.3923) -> (-60.6687, 62.8923)
  line L746 (-60.6687, 62.8923) -> (-60.6687, 67.8923)
  line L747 (-60.6687, 67.8923) -> (-64.9988, 70.3923)
  line L748 (-54.3385, 70.3923) -> (-58.6687, 67.8923)
  line L749 (-58.6687, 67.8923) -> (-58.6687, 62.8923)
  line L750 (-58.6687, 62.8923) -> (-54.3385, 60.3923)
  line L751 (-54.3385, 60.3923) -> (-50.0084, 62.8923)
  line L752 (-50.0084, 62.8923) -> (-50.0084, 67.8923)
  line L753 (-50.0084, 67.8923) -> (-54.3385, 70.3923)
  line L754 (-43.6783, 70.3923) -> (-48.0084, 67.8923)
  line L755 (-48.0084, 67.8923) -> (-48.0084, 62.8923)
  line L756 (-48.0084, 62.8923) -> (-43.6783, 60.3923)
  line L757 (-43.6783, 60.3923) -> (-39.3482, 62.8923)
  line L758 (-39.3482, 62.8923) -> (-39.3482, 67.8923)
  line L759 (-39.3482, 67.8923) -> (-43.6783, 70.3923)
  line L760 (-33.018, 70.3923) -> (-37.3482, 67.8923)
  line L761 (-37.3482, 67.8923) -> (-37.3482, 62.8923)
  line L762 (-37.3482, 62.8923) -> (-33.018, 60.3923)
  line L763 (-33.018, 60.3923) -> (-28.6879, 62.8923)
  line L764 (-28.6879, 62.8923) -> (-28.6879, 67.8923)
  line L765 (-28.6879, 67.8923) -> (-33.018, 70.3923)
  line L766 (-22.3578, 70.3923) -> (-26.6879, 67.8923)
  line L767 (-26.6879, 67.8923) -> (-26.6879, 62.8923)
  line L768 (-26.6879, 62.8923) -> (-22.3578, 60.3923)
  line L769 (-22.3578, 60.3923) -> (-18.0277, 62.8923)
  line L770 (-18.0277, 62.8923) -> (-18.0277, 67.8923)
  line L771 (-18.0277, 67.8923) -> (-22.3578, 70.3923)
  line L772 (-11.6975, 70.3923) -> (-16.0277, 67.8923)
  line L773 (-16.0277, 67.8923) -> (-16.0277, 62.8923)
  line L774 (-16.0277, 62.8923) -> (-11.6975, 60.3923)
  line L775 (-11.6975, 60.3923) -> (-7.3674, 62.8923)
  line L776 (-7.3674, 62.8923) -> (-7.3674, 67.8923)
  line L777 (-7.3674, 67.8923) -> (-11.6975, 70.3923)
  line L778 (-1.0373, 70.3923) -> (-5.3674, 67.8923)
  line L779 (-5.3674, 67.8923) -> (-5.3674, 62.8923)
  line L780 (-5.3674, 62.8923) -> (-1.0373, 60.3923)
  line L781 (-1.0373, 60.3923) -> (3.2929, 62.8923)
  line L782 (3.2929, 62.8923) -> (3.2929, 67.8923)
  line L783 (3.2929, 67.8923) -> (-1.0373, 70.3923)
  line L784 (9.623, 70.3923) -> (5.2929, 67.8923)
  line L785 (5.2929, 67.8923) -> (5.2929, 62.8923)
  line L786 (5.2929, 62.8923) -> (9.623, 60.3923)
  line L787 (9.623, 60.3923) -> (13.9531, 62.8923)
  line L788 (13.9531, 62.8923) -> (13.9531, 67.8923)
  line L789 (13.9531, 67.8923) -> (9.623, 70.3923)
  line L790 (20.2832, 70.3923) -> (15.9531, 67.8923)
  line L791 (15.9531, 67.8923) -> (15.9531, 62.8923)
  line L792 (15.9531, 62.8923) -> (20.2832, 60.3923)
  line L793 (20.2832, 60.3923) -> (24.6134, 62.8923)
  line L794 (24.6134, 62.8923) -> (24.6134, 67.8923)
  line L795 (24.6134, 67.8923) -> (20.2832, 70.3923)
  line L796 (30.9435, 70.3923) -> (26.6134, 67.8923)
  line L797 (26.6134, 67.8923) -> (26.6134, 62.8923)
  line L798 (26.6134, 62.8923) -> (30.9435, 60.3923)
  line L799 (30.9435, 60.3923) -> (35.2736, 62.8923)
  line L800 (35.2736, 62.8923) -> (35.2736, 67.8923)
  line L801 (35.2736, 67.8923) -> (30.9435, 70.3923)
  line L802 (41.6037, 70.3923) -> (37.2736, 67.8923)
  line L803 (37.2736, 67.8923) -> (37.2736, 62.8923)
  line L804 (37.2736, 62.8923) -> (41.6037, 60.3923)
  line L805 (41.6037, 60.3923) -> (45.9339, 62.8923)
  line L806 (45.9339, 62.8923) -> (45.9339, 67.8923)
  line L807 (45.9339, 67.8923) -> (41.6037, 70.3923)
  line L808 (52.264, 70.3923) -> (47.9339, 67.8923)
  line L809 (47.9339, 67.8923) -> (47.9339, 62.8923)
  line L810 (47.9339, 62.8923) -> (52.264, 60.3923)
  line L811 (52.264, 60.3923) -> (56.5941, 62.8923)
  line L812 (56.5941, 62.8923) -> (56.5941, 67.8923)
  line L813 (56.5941, 67.8923) -> (52.264, 70.3923)
  line L814 (62.9242, 70.3923) -> (58.5941, 67.8923)
  line L815 (58.5941, 67.8923) -> (58.5941, 62.8923)
  line L816 (58.5941, 62.8923) -> (62.9242, 60.3923)
  line L817 (62.9242, 60.3923) -> (67.2544, 62.8923)
  line L818 (67.2544, 62.8923) -> (67.2544, 67.8923)
  line L819 (67.2544, 67.8923) -> (62.9242, 70.3923)
  line L820 (73.5845, 70.3923) -> (69.2544, 67.8923)
  line L821 (69.2544, 67.8923) -> (69.2544, 62.8923)
  line L822 (69.2544, 62.8923) -> (73.5845, 60.3923)
  line L823 (73.5845, 60.3923) -> (77.9146, 62.8923)
  line L824 (77.9146, 62.8923) -> (77.9146, 67.8923)
  line L825 (77.9146, 67.8923) -> (73.5845, 70.3923)
  line L826 (84.2448, 70.3923) -> (79.9146, 67.8923)
  line L827 (79.9146, 67.8923) -> (79.9146, 62.8923)
  line L828 (79.9146, 62.8923) -> (84.2448, 60.3923)
  line L829 (84.2448, 60.3923) -> (88.5749, 62.8923)
  line L830 (88.5749, 62.8923) -> (88.5749, 67.8923)
  line L831 (88.5749, 67.8923) -> (84.2448, 70.3923)
  line L832 (94.905, 70.3923) -> (90.5749, 67.8923)
  line L833 (90.5749, 67.8923) -> (90.5749, 62.8923)
  line L834 (90.5749, 62.8923) -> (94.905, 60.3923)
  line L835 (94.905, 60.3923) -> (99.2351, 62.8923)
  line L836 (99.2351, 62.8923) -> (99.2351, 67.8923)
  line L837 (99.2351, 67.8923) -> (94.905, 70.3923)
  line L838 (105.5653, 70.3923) -> (101.2351, 67.8923)
  line L839 (101.2351, 67.8923) -> (101.2351, 62.8923)
  line L840 (101.2351, 62.8923) -> (105.5653, 60.3923)
  line L841 (105.5653, 60.3923) -> (109.8954, 62.8923)
  line L842 (109.8954, 62.8923) -> (109.8954, 67.8923)
  line L843 (109.8954, 67.8923) -> (105.5653, 70.3923)
  line L844 (116.2255, 70.3923) -> (111.8954, 67.8923)
  line L845 (111.8954, 67.8923) -> (111.8954, 62.8923)
  line L846 (111.8954, 62.8923) -> (116.2255, 60.3923)
  line L847 (116.2255, 60.3923) -> (120.5556, 62.8923)
  line L848 (120.5556, 62.8923) -> (120.5556, 67.8923)
  line L849 (120.5556, 67.8923) -> (116.2255, 70.3923)
  line L850 (126.8858, 70.3923) -> (122.5556, 67.8923)
  line L851 (122.5556, 67.8923) -> (122.5556, 62.8923)
  line L852 (122.5556, 62.8923) -> (126.8858, 60.3923)
  line L853 (126.8858, 60.3923) -> (131.2159, 62.8923)
  line L854 (131.2159, 62.8923) -> (131.2159, 67.8923)
  line L855 (131.2159, 67.8923) -> (126.8858, 70.3923)
  line L856 (137.546, 70.3923) -> (133.2159, 67.8923)
  line L857 (133.2159, 67.8923) -> (133.2159, 62.8923)
  line L858 (133.2159, 62.8923) -> (137.546, 60.3923)
  line L859 (137.546, 60.3923) -> (141.8762, 62.8923)
  line L860 (141.8762, 62.8923) -> (141.8762, 67.8923)
  line L861 (141.8762, 67.8923) -> (137.546, 70.3923)
  line L862 (148.2063, 70.3923) -> (143.8762, 67.8923)
  line L863 (143.8762, 67.8923) -> (143.8762, 62.8923)
  line L864 (143.8762, 62.8923) -> (148.2063, 60.3923)
  line L865 (148.2063, 60.3923) -> (152.5364, 62.8923)
  line L866 (152.5364, 62.8923) -> (152.5364, 67.8923)
  line L867 (152.5364, 67.8923) -> (148.2063, 70.3923)
  line L868 (-59.6687, 79.6244) -> (-63.9988, 77.1244)
  line L869 (-63.9988, 77.1244) -> (-63.9988, 72.1244)
  line L870 (-63.9988, 72.1244) -> (-59.6687, 69.6244)
  line L871 (-59.6687, 69.6244) -> (-55.3385, 72.1244)
  line L872 (-55.3385, 72.1244) -> (-55.3385, 77.1244)
  line L873 (-55.3385, 77.1244) -> (-59.6687, 79.6244)
  line L874 (-49.0084, 79.6244) -> (-53.3385, 77.1244)
  line L875 (-53.3385, 77.1244) -> (-53.3385, 72.1244)
  line L876 (-53.3385, 72.1244) -> (-49.0084, 69.6244)
  line L877 (-49.0084, 69.6244) -> (-44.6783, 72.1244)
  line L878 (-44.6783, 72.1244) -> (-44.6783, 77.1244)
  line L879 (-44.6783, 77.1244) -> (-49.0084, 79.6244)
  line L880 (-38.3482, 79.6244) -> (-42.6783, 77.1244)
  line L881 (-42.6783, 77.1244) -> (-42.6783, 72.1244)
  line L882 (-42.6783, 72.1244) -> (-38.3482, 69.6244)
  line L883 (-38.3482, 69.6244) -> (-34.018, 72.1244)
  line L884 (-34.018, 72.1244) -> (-34.018, 77.1244)
  line L885 (-34.018, 77.1244) -> (-38.3482, 79.6244)
  line L886 (-27.6879, 79.6244) -> (-32.018, 77.1244)
  line L887 (-32.018, 77.1244) -> (-32.018, 72.1244)
  line L888 (-32.018, 72.1244) -> (-27.6879, 69.6244)
  line L889 (-27.6879, 69.6244) -> (-23.3578, 72.1244)
  line L890 (-23.3578, 72.1244) -> (-23.3578, 77.1244)
  line L891 (-23.3578, 77.1244) -> (-27.6879, 79.6244)
  line L892 (-17.0277, 79.6244) -> (-21.3578, 77.1244)
  line L893 (-21.3578, 77.1244) -> (-21.3578, 72.1244)
  line L894 (-21.3578, 72.1244) -> (-17.0277, 69.6244)
  line L895 (-17.0277, 69.6244) -> (-12.6975, 72.1244)
  line L896 (-12.6975, 72.1244) -> (-12.6975, 77.1244)
  line L897 (-12.6975, 77.1244) -> (-17.0277, 79.6244)
  line L898 (-6.3674, 79.6244) -> (-10.6975, 77.1244)
  line L899 (-10.6975, 77.1244) -> (-10.6975, 72.1244)
  line L900 (-10.6975, 72.1244) -> (-6.3674, 69.6244)
  line L901 (-6.3674, 69.6244) -> (-2.0373, 72.1244)
  line L902 (-2.0373, 72.1244) -> (-2.0373, 77.1244)
  line L903 (-2.0373, 77.1244) -> (-6.3674, 79.6244)
  line L904 (4.2929, 79.6244) -> (-0.0373, 77.1244)
  line L905 (-0.0373, 77.1244) -> (-0.0373, 72.1244)
  line L906 (-0.0373, 72.1244) -> (4.2929, 69.6244)
  line L907 (4.2929, 69.6244) -> (8.623, 72.1244)
  line L908 (8.623, 72.1244) -> (8.623, 77.1244)
  line L909 (8.623, 77.1244) -> (4.2929, 79.6244)
  line L910 (14.9531, 79.6244) -> (10.623, 77.1244)
  line L911 (10.623, 77.1244) -> (10.623, 72.1244)
  line L912 (10.623, 72.1244) -> (14.9531, 69.6244)
  line L913 (14.9531, 69.6244) -> (19.2832, 72.1244)
  line L914 (19.2832, 72.1244) -> (19.2832, 77.1244)
  line L915 (19.2832, 77.1244) -> (14.9531, 79.6244)
  line L916 (25.6134, 79.6244) -> (21.2832, 77.1244)
  line L917 (21.2832, 77.1244) -> (21.2832, 72.1244)
  line L918 (21.2832, 72.1244) -> (25.6134, 69.6244)
  line L919 (25.6134, 69.6244) -> (29.9435, 72.1244)
  line L920 (29.9435, 72.1244) -> (29.9435, 77.1244)
  line L921 (29.9435, 77.1244) -> (25.6134, 79.6244)
  line L922 (36.2736, 79.6244) -> (31.9435, 77.1244)
  line L923 (31.9435, 77.1244) -> (31.9435, 72.1244)
  line L924 (31.9435, 72.1244) -> (36.2736, 69.6244)
  line L925 (36.2736, 69.6244) -> (40.6037, 72.1244)
  line L926 (40.6037, 72.1244) -> (40.6037, 77.1244)
  line L927 (40.6037, 77.1244) -> (36.2736, 79.6244)
  line L928 (46.9339, 79.6244) -> (42.6037, 77.1244)
  line L929 (42.6037, 77.1244) -> (42.6037, 72.1244)
  line L930 (42.6037, 72.1244) -> (46.9339, 69.6244)
  line L931 (46.9339, 69.6244) -> (51.264, 72.1244)
  line L932 (51.264, 72.1244) -> (51.264, 77.1244)
  line L933 (51.264, 77.1244) -> (46.9339, 79.6244)
  line L934 (57.5941, 79.6244) -> (53.264, 77.1244)
  line L935 (53.264, 77.1244) -> (53.264, 72.1244)
  line L936 (53.264, 72.1244) -> (57.5941, 69.6244)
  line L937 (57.5941, 69.6244) -> (61.9242, 72.1244)
  line L938 (61.9242, 72.1244) -> (61.9242, 77.1244)
  line L939 (61.9242, 77.1244) -> (57.5941, 79.6244)
  line L940 (68.2544, 79.6244) -> (63.9242, 77.1244)
  line L941 (63.9242, 77.1244) -> (63.9242, 72.1244)
  line L942 (63.9242, 72.1244) -> (68.2544, 69.6244)
  line L943 (68.2544, 69.6244) -> (72.5845, 72.1244)
  line L944 (72.5845, 72.1244) -> (72.5845, 77.1244)
  line L945 (72.5845, 77.1244) -> (68.2544, 79.6244)
  line L946 (78.9146, 79.6244) -> (74.5845, 77.1244)
  line L947 (74.5845, 77.1244) -> (74.5845, 72.1244)
  line L948 (74.5845, 72.1244) -> (78.9146, 69.6244)
  line L949 (78.9146, 69.6244) -> (83.2448, 72.1244)